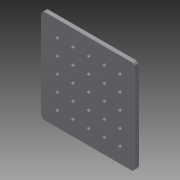
# Autodesk Inventor part: 5x5x5 solder helper
Saved by Autodesk Inventor 2015 (Build 190159000, 159)
## iProperties
Created: 2016-02-20
Part Number: 5x5x5 solder helper
Material: Generic
Document SubType Name: Modeling
Designer: william
Density: 1 g/cm^3
Appearance: Default
Author: william
Autodesk Inventor part; units mm, degrees
ref_plane "YZ Plane" through (0, 0, 0) normal (1, 0, 0) x (0, 1, 0)
ref_plane "XZ Plane" through (0, 0, 0) normal (0, 1, 0) x (-1, 0, 0)
ref_plane "XY Plane" through (0, 0, 0) normal (0, 0, 1) x (1, 0, 0)
sketch "Sketch1" plane through (0, 0, 0) normal (0, 1, 0) x (-1, 0, 0)
  line L0 (0, 0) -> (-120, 0)
  line L1 (-120, 0) -> (-120, -120)
  line L2 (-120, -120) -> (0, -120)
  line L3 (0, -120) -> (0, 0)
  circle A0 centre (-20, -20) radius 2.5
  circle A1 centre (-40, -20) radius 2.5
  circle A2 centre (-60, -20) radius 2.5
  circle A3 centre (-80, -20) radius 2.5
  circle A4 centre (-100, -20) radius 2.5
  circle A5 centre (-20, -40) radius 2.5
  circle A6 centre (-40, -40) radius 2.5
  circle A7 centre (-60, -40) radius 2.5
  circle A8 centre (-80, -40) radius 2.5
  circle A9 centre (-100, -40) radius 2.5
  circle A10 centre (-20, -60) radius 2.5
  circle A11 centre (-40, -60) radius 2.5
  circle A12 centre (-60, -60) radius 2.5
  circle A13 centre (-80, -60) radius 2.5
  circle A14 centre (-100, -60) radius 2.5
  circle A15 centre (-20, -80) radius 2.5
  circle A16 centre (-40, -80) radius 2.5
  circle A17 centre (-60, -80) radius 2.5
  circle A18 centre (-80, -80) radius 2.5
  circle A19 centre (-100, -80) radius 2.5
  circle A20 centre (-20, -100) radius 2.5
  circle A21 centre (-40, -100) radius 2.5
  circle A22 centre (-60, -100) radius 2.5
  circle A23 centre (-80, -100) radius 2.5
  circle A24 centre (-100, -100) radius 2.5
  dimension "d0" = 120
  dimension "d1" = 120
  dimension "d2" = 5
  dimension "d4" = 20
  dimension "d5" = 20
  dimension "d8" = 20
  dimension "d11" = 20
  constraints: 25 centre point, 8 end point, 2 horizontal, 2 parallel, 1 perpendicular, 1 vertical, 48 other
  measures "d0" distance of L1.end L2.end
  measures "d1" distance of L0.end L1.end
  measures "d2" diameter of A0
  measures "d4" distance from line of A0.centre L0
  measures "d5" distance from line of A0.centre L3
  measures "d8" distance of A0.centre A1.centre
  measures "d11" distance of A0.centre A5.centre
extrude "Extrusion1" add sketch "Sketch1" along normal blind 5
fillet "Fillet1" radius 5 4 edges at (0, 2.5, -120) (0, 2.5, 0) (120, 2.5, 0) (120, 2.5, -120)
body "Solid1"
